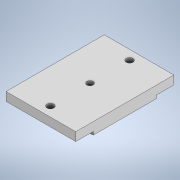
# Autodesk Inventor part: EOM mount
Saved by Autodesk Inventor 2020 (Build 240168000, 168)
## iProperties
Created: 2020-10-29
Part Number: EOM mount
Material: Generic
Document SubType Name: Modeling
Designer: Austin
Density: 1 g/cm^3
Appearance: Default
Author: Austin
Autodesk Inventor part; units mm, degrees
ref_plane "YZ Plane" through (0, 0, 0) normal (1, 0, 0) x (0, 1, 0)
ref_plane "XZ Plane" through (0, 0, 0) normal (0, 1, 0) x (-1, 0, 0)
ref_plane "XY Plane" through (0, 0, 0) normal (0, 0, 1) x (1, 0, 0)
sketch "Sketch1" plane through (0, 0, 0) normal (0, 1, 0) x (-1, 0, 0)
  line L0 (22, 20) -> (-22, 20)
  line L1 (-22, 20) -> (-22, -20)
  line L2 (-22, -20) -> (22, -20)
  line L3 (22, -20) -> (22, 20)
  line L4 (22, 20) -> (-22, -20) construction
  line L5 (-22, 20) -> (22, -20) construction
  point P0 (0, 0)
  dimension "CUBE_DIM" = 40
  dimension "d1" = 44
  constraints: 12 end point, 2 midpoint, 2 parallel, 1 horizontal, 1 perpendicular
  measures "CUBE_DIM" distance of L2.end L0.start
  measures "d1" distance of L1.end L2.end
extrude "Extrusion1" add sketch "Sketch1" along normal blind 5.4
sketch "Sketch2" plane through (0, 5.4, 0) normal (0, 1, 0) x (1, 0, 0)
  line L0 (-22, -31) -> (22, -31)
  line L1 (22, -31) -> (22, 31)
  line L2 (22, 31) -> (-22, 31)
  line L3 (-22, 31) -> (-22, -31)
  line L4 (-22, -31) -> (22, 31) construction
  line L5 (22, -31) -> (-22, 31) construction
  line L6 (-22, 20) -> (-22, -20) projected
  line L7 (-22, -20) -> (22, -20)
  line L8 (22, 20) -> (-22, 20) projected
  line L9 (-22, 20) -> (22, 20)
  point P0 (0, 0)
  dimension "BASE_LENGTH" = 62
  dimension "BASE_WIDTH" = 44
  constraints: 16 end point, 3 equal length, 2 midpoint, 2 perpendicular, 1 horizontal, 1 point on line
  measures "BASE_LENGTH" distance of L2.end L0.start
  measures "BASE_WIDTH" distance of L0.start L0.end
extrude "Extrusion2" add sketch "Sketch2" against normal blind 5.4
sketch "Sketch5" plane through (0, 0, 0) normal (0, -1, 0) x (1, 0, 0)
  line L0 (22, 20) -> (20, 20)
  line L1 (20, 20) -> (20, -20)
  line L2 (20, -20) -> (22, -20)
  line L3 (22, -20) -> (22, 20)
  line L4 (22, 31) -> (22, -31) projected
  point P0 (0, 0)
  dimension "d31" = 40
  dimension "d32" = 20
  dimension "d33" = 0
  dimension "d34" = 2
  constraints: 8 end point, 2 parallel, 1 horizontal, 1 perpendicular
  measures "d31" distance of L2.end L0.start
  measures "d32" distance from line of point (0, 0) L2
  measures "d33" distance between parallel lines of L4 L3
  measures "d34" distance of L1.end L2.end
extrude "Extrusion3" add sketch "Sketch5" along normal blind 2
sketch "Sketch3" plane through (0, 5.4, 0) normal (0, 1, 0) x (1, 0, 0)
  circle A0 centre (0, 0) radius 2.9522
  line L0 (20, 20) -> (20, -20) projected
  dimension "d35" = 20
  constraints: 1 centre point, 1 coincident
  measures "d35" distance from line of L0 A0.centre
hole "Hole1" at (0, 5.4, 0) direction (0, -1, 0) diameter 3.242 depth 5.4 counterbore diameter 4 counterbore depth 1.9 thread size "M4x0.7" class "6H" standard "ANSI Metric M Profile"
sketch "Sketch4" plane through (0, 0, 0) normal (0, -1, 0) x (1, 0, 0)
  circle A0 centre (0, -25) radius 1.0924
  circle A1 centre (0, 25) radius 1.3036
  line L0 (-22, -31) -> (22, -31) projected
  line L1 (22, 31) -> (-22, 31) projected
  point P0 (0, 0)
  point P1 (-22, -29)
  point P2 (-22, 29)
  point P3 (22, -31)
  point P4 (-22, 31)
  dimension "d22" = 6
  dimension "d23" = 6
  constraints: 2 centre point, 2 other
hole "Hole2" at (0, 0, 25) at (0, 0, -25) direction (0, 1, 0) diameter 4.31 depth 12.3 counterbore diameter 7.94 counterbore depth 2.4 clearance for "Socket Head Cap Screw" size "#8" standard "Ansi Unified Screw Threads"
equation "\"PLATFORM_HEIGHT\" = BEAM_HEIGHT - 0.5 * CUBE_DIM"
equation "\"BASE_LENGTH\" = CUBE_DIM + 2 * WING_SIZE"
equation "\"d32\" = 0.5 * d31"
equation "\"d13\" = PLATFORM_HEIGHT"
equation "\"WING_SIZE\" = 11"
equation "\"BEAM_HEIGHT\" = 25.4"
body "Solid1"
